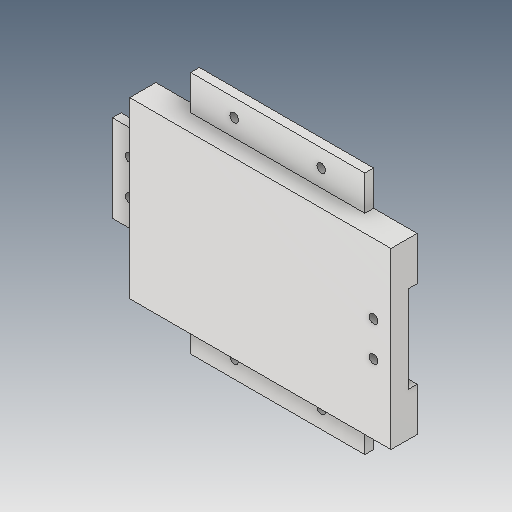
# Autodesk Inventor part: CP007
Saved by Autodesk Inventor 2017 (Build 210142000, 142)
## iProperties
Created: 2017-05-15
Part Number: CP007
Material: ABS Plastic
Document SubType Name: Modeling
Designer: zallen
Density: 1.06 g/cm^3
Appearance: Smooth - White
Mass: 258.659 g
Surface Area: 487.712 cm^2
Volume: 244.018 cm^3
Author: zallen
Autodesk Inventor part; units mm, degrees
ref_plane "YZ Plane" through (0, 0, 0) normal (1, 0, 0) x (0, 1, 0)
ref_plane "XZ Plane" through (0, 0, 0) normal (0, 1, 0) x (-1, 0, 0)
ref_plane "XY Plane" through (0, 0, 0) normal (0, 0, 1) x (1, 0, 0)
sketch "Sketch1" plane through (0, 0, 0) normal (0, 0, 1) x (1, 0, 0)
  line L0 (0, 0) -> (150, 0)
  line L1 (150, 0) -> (150, 100)
  line L2 (150, 100) -> (0, 100)
  line L3 (0, 100) -> (0, 0)
  dimension "d0" = 150
  dimension "d1" = 100
  constraints: 8 end point, 2 parallel, 1 horizontal, 1 perpendicular
  measures "d0" distance of L2.end L1.end
  measures "d1" distance of L1.end L0.end
extrude "Extrusion1" add sketch "Sketch1" along normal blind 15
sketch "Sketch7" plane through (0, 0, 0) normal (0, 0, -1) x (-1, 0, 0)
  line L0 (0, 25) -> (20, 25)
  line L1 (20, 25) -> (20, 75)
  line L2 (20, 75) -> (0, 75)
  line L3 (0, 75) -> (0, 25)
  point P0 (0, 0)
  dimension "d27" = 20
  dimension "d28" = 50
  dimension "d29" = 25
  constraints: 8 end point, 2 parallel, 1 horizontal, 1 perpendicular
  measures "d27" distance of L2.end L1.end
  measures "d28" distance of L1.end L0.end
  measures "d29" distance of point (0, 0) L0.start
extrude "Extrusion7" add sketch "Sketch7" against normal blind 5
sketch "Sketch8" plane through (0, 0, 0) normal (0, 0, -1) x (-1, 0, 0)
  line L0 (-25, 0) -> (-125, 0)
  line L1 (-125, 0) -> (-125, -20)
  line L2 (-125, -20) -> (-25, -20)
  line L3 (-25, -20) -> (-25, 0)
  line L4 (-150, 100) -> (0, 100) projected
  line L5 (-25, 100) -> (-125, 100)
  line L6 (-125, 100) -> (-125, 120)
  line L7 (-125, 120) -> (-25, 120)
  line L8 (-25, 120) -> (-25, 100)
  point P0 (0, 0)
  dimension "d32" = 100
  dimension "d33" = 20
  dimension "d34" = 25
  dimension "d37" = 100
  dimension "d38" = 20
  constraints: 16 end point, 4 parallel, 2 horizontal, 2 perpendicular, 1 point on line
  measures "d32" distance of L2.end L1.end
  measures "d33" distance of L1.end L0.end
  measures "d34" distance of L0.start point (0, 0)
  measures "d37" distance of L6.end L7.end
  measures "d38" distance of L5.end L6.end
extrude "Extrusion8" add sketch "Sketch8" against normal blind 5
sketch "Sketch9" plane through (0, 0, 0) normal (0, 0, -1) x (-1, 0, 0)
  circle A0 centre (-50, -10) radius 2.5
  circle A1 centre (-100, -10) radius 2.5
  line L0 (-25, -20) -> (-25, 0) projected
  line L1 (-125, 0) -> (-125, -20) projected
  line L2 (-25, 0) -> (-125, 0) projected
  circle A2 centre (-50, 110) radius 2.5
  circle A3 centre (-100, 110) radius 2.5
  line L3 (-125, 120) -> (-25, 120) projected
  circle A4 centre (10, 40) radius 2.5
  circle A5 centre (10, 60) radius 2.5
  line L4 (0, 75) -> (0, 25) projected
  line L5 (0, 25) -> (20, 25) projected
  line L6 (20, 75) -> (0, 75) projected
  point P0 (0, 0)
  dimension "d39" = 5
  dimension "d40" = 5
  dimension "d41" = 25
  dimension "d42" = 25
  dimension "d43" = 10
  dimension "d44" = 5
  dimension "d45" = 5
  dimension "d46" = 10
  dimension "d47" = 5
  dimension "d48" = 5
  dimension "d49" = 10
  dimension "d50" = 15
  dimension "d51" = 15
  constraints: 6 centre point, 3 vertical alignment, 2 horizontal alignment
  measures "d39" diameter of A0
  measures "d40" diameter of A1
  measures "d41" distance from line of L0 A0.centre
  measures "d42" distance from line of L1 A1.centre
  measures "d43" distance from line of L2 A0.centre
  measures "d44" diameter of A2
  measures "d45" diameter of A3
  measures "d46" distance from line of L3 A2.centre
  measures "d47" diameter of A4
  measures "d48" diameter of A5
  measures "d49" distance from line of L4 A4.centre
  measures "d50" distance from line of L5 A4.centre
  measures "d51" distance from line of L6 A5.centre
extrude "Extrusion9" cut sketch "Sketch9" against normal through all
thread "Thread1" size "M5x0.8" class "6H" standard "ANSI Metric M Profile" full length
thread "Thread2" size "M5x0.8" class "6H" standard "ANSI Metric M Profile" full length
thread "Thread3" size "M5x0.8" class "6H" standard "ANSI Metric M Profile" full length
thread "Thread4" size "M5x0.8" class "6H" standard "ANSI Metric M Profile" full length
thread "Thread5" size "M5x0.8" class "6H" standard "ANSI Metric M Profile" full length
thread "Thread6" size "M5x0.8" class "6H" standard "ANSI Metric M Profile" full length
sketch "Sketch10" plane through (0, 0, 0) normal (0, 0, -1) x (-1, 0, 0)
  line L0 (-150, 0) -> (-150, 100) projected
  line L1 (-150, 25) -> (-130, 25)
  line L2 (-130, 25) -> (-130, 75)
  line L3 (-130, 75) -> (-150, 75)
  line L4 (-150, 75) -> (-150, 25)
  circle A0 centre (10, 40) radius 2.5 projected
  circle A1 centre (-50, 110) radius 2.5 projected
  circle A2 centre (-50, -10) radius 2.5 projected
  circle A3 centre (-100, -10) radius 2.5 projected
  circle A4 centre (-100, 110) radius 2.5 projected
  circle A5 centre (10, 60) radius 2.5 projected
  line L5 (0, 0) -> (-25, 0) projected
  line L6 (0, 25) -> (0, 0) projected
  line L7 (0, 25) -> (20, 25) projected
  line L8 (20, 25) -> (20, 75) projected
  line L9 (20, 75) -> (0, 75) projected
  line L10 (0, 100) -> (0, 75) projected
  line L11 (-25, 100) -> (0, 100) projected
  line L12 (-25, 120) -> (-25, 100) projected
  line L13 (-125, 120) -> (-25, 120) projected
  line L14 (-125, 100) -> (-125, 120) projected
  line L15 (-150, 100) -> (-125, 100) projected
  line L16 (-150, 0) -> (-150, 100) projected
  line L17 (-125, 0) -> (-150, 0) projected
  line L18 (-125, 0) -> (-125, -20) projected
  line L19 (-125, -20) -> (-25, -20) projected
  line L20 (-25, -20) -> (-25, 0) projected
  dimension "d66" = 20
  dimension "d67" = 50
  constraints: 8 end point, 2 parallel, 1 horizontal, 1 horizontal alignment, 1 perpendicular, 1 point on line
  measures "d66" distance of L3.end L2.end
  measures "d67" distance of L2.end L1.end
extrude "Extrusion10" cut sketch "Sketch10" against normal blind 5 contours L0 L3 L2 L1
sketch "Sketch11" plane through (0, 0, 5) normal (0, 0, -1) x (-1, 0, 0)
  circle A0 centre (-140, 60) radius 2.5
  circle A1 centre (-140, 40) radius 2.5
  line L0 (-130, 25) -> (-150, 25) projected
  line L1 (-150, 0) -> (-150, 25) projected
  line L2 (-125, 0) -> (-150, 0) projected
  line L3 (-125, 0) -> (-125, -20) projected
  line L4 (-125, -20) -> (-25, -20) projected
  line L5 (-25, -20) -> (-25, 0) projected
  line L6 (0, 0) -> (-25, 0) projected
  line L7 (0, 25) -> (0, 0) projected
  line L8 (0, 25) -> (20, 25) projected
  line L9 (20, 25) -> (20, 75) projected
  line L10 (20, 75) -> (0, 75) projected
  line L11 (0, 100) -> (0, 75) projected
  line L12 (-25, 100) -> (0, 100) projected
  line L13 (-25, 120) -> (-25, 100) projected
  line L14 (-125, 120) -> (-25, 120) projected
  line L15 (-125, 100) -> (-125, 120) projected
  line L16 (-150, 100) -> (-125, 100) projected
  line L17 (-150, 75) -> (-150, 100) projected
  line L18 (-150, 75) -> (-130, 75) projected
  line L19 (-130, 75) -> (-130, 25) projected
  circle A2 centre (10, 40) radius 2.5 projected
  circle A3 centre (-50, 110) radius 2.5 projected
  circle A4 centre (-50, -10) radius 2.5 projected
  circle A5 centre (-100, -10) radius 2.5 projected
  circle A6 centre (-100, 110) radius 2.5 projected
  circle A7 centre (10, 60) radius 2.5 projected
  line L20 (-150, 25) -> (-150, 75) projected
  dimension "d70" = 5
  dimension "d71" = 5
  dimension "d72" = 10
  dimension "d79" = 15
  constraints: 2 centre point, 1 horizontal alignment, 1 vertical alignment
  measures "d70" diameter of A0
  measures "d71" diameter of A1
  measures "d72" distance from line of L20 A1.centre
  measures "d79" distance from line of L0 A1.centre
extrude "Extrusion11" cut sketch "Sketch11" against normal through all contours A0 | A1
thread "Thread7" size "M5x0.8" class "6H" standard "ANSI Metric M Profile" full length
thread "Thread8" size "M5x0.8" class "6H" standard "ANSI Metric M Profile" full length
body "Solid1"
